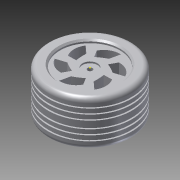
# Autodesk Inventor part: Wheels1
Saved by Autodesk Inventor 2015 (Build 190159000, 159)
## iProperties
Created: 2014-11-04
Part Number: Wheels1
Material: ABS Plastic
Document SubType Name: Modeling
Designer: ah14592
Density: 1.06 g/cm^3
Appearance: Smooth - White
Author: ah14592
Autodesk Inventor part; units mm, degrees
ref_plane "YZ Plane" through (0, 0, 0) normal (1, 0, 0) x (0, 1, 0)
ref_plane "XZ Plane" through (0, 0, 0) normal (0, 1, 0) x (-1, 0, 0)
sketch "Sketch1" plane through (0, 0, 0) normal (0, 1, 0) x (-1, 0, 0)
  line L0 (0, 0) -> (0, 48.3347) construction
  line L1 (-23, 44.2835) -> (-28, 44.2835)
  line L2 (-28, 44.2835) -> (-28, 14.2835)
  line L3 (-28, 14.2835) -> (-23, 14.2835)
  line L4 (-23, 14.2835) -> (-23, 44.2835)
  point P0 (0, 23.2008)
  dimension "d2" = 5
  dimension "d3" = 30
  dimension "d4" = 23
  constraints: 10 end point, 2 parallel, 2 vertical, 1 horizontal, 1 perpendicular, 1 point on line
  measures "d2" distance of L3.end L2.end
  measures "d3" distance of L2.end L1.end
  measures "d4" distance between parallel lines of L4 L0
revolve "Revolution1" add sketch "Sketch1" angle 360 about axis through (0, 0, 0) along (0, 0, 1)
sketch "Sketch7" plane through (0, 0, 44.2835) normal (0, 0, 1) x (1, 0, 0)
  circle A0 centre (0, 0) radius 24
  dimension "d33" = 48
  constraints: 1 centre point, 1 coincident
  measures "d33" diameter of A0
extrude "Extrusion4" add sketch "Sketch7" against normal blind 13
fillet "Fillet4" radius 3 2 edges at (-28, 0, 44.2835) (-28, 0, 14.2835)
sketch "Sketch8" plane through (0, 0, 44.2835) normal (0, 0, 1) x (1, 0, 0)
  circle A0 centre (0, 0) radius 23 projected
  circle A1 centre (0, 0) radius 25 projected
  circle A2 centre (0, 0) radius 28 projected
  circle A3 centre (0, 0) radius 25 projected
  circle A4 centre (0, 0) radius 23
  constraints: 1 centre point, 1 coincident, 1 concentric
fillet "Fillet5" radius 3 1 edges at (-23, 0, 31.2835)
sketch "Sketch9" plane through (0, 0, 44.2835) normal (0, 0, 1) x (1, 0, 0)
  circle A0 centre (0, 0) radius 23 projected
  circle A1 centre (0, 0) radius 20 projected
  circle A2 centre (0, 0) radius 20
  constraints: 1 centre point, 1 coincident, 1 concentric
extrude "Extrusion5" cut sketch "Sketch9" against normal blind 2 contours A1
chamfer "Chamfer1" distance 1 angle 45 1 edges at (-20, 0, 44.2835)
sketch "Sketch10" plane through (0, 0, 42.2835) normal (0, 0, 1) x (1, 0, 0)
  line L0 (-16.9268, -6.6619) -> (-10.5367, -4.6226)
  line L1 (-6.7299, -12.6441) -> (-4.1467, -7.8856)
  arc A0 (-16.9268, -6.6619) -> (-6.7299, -12.6441) centre (-7.1975, -1.7595) ccw
  arc A1 (-10.5367, -4.6226) -> (-4.1467, -7.8856) centre (7.1055, 22.0383) ccw
  point P0 (0, 0)
  constraints: 4 end point, 4 point on circle, 2 centre point
extrude "Extrusion6" cut sketch "Sketch10" against normal through all
pattern_circular "Circular Pattern2" count 6 over 360 about axis through (0, 0, -10) along (0, 0, 1) of "Extrusion6"
sketch "Sketch11" plane through (0, 0, 42.2835) normal (0, 0, 1) x (1, 0, 0)
  point P0 (0, 0)
hole "Hole3" at (0, 0, 44.2835) direction (0, 0, -1) diameter 3.2 end through all counterbore diameter 10 counterbore depth 3
sketch "Sketch12" plane through (0, 0, 31.2835) normal (0, 0, -1) x (-1, 0, 0)
  point P0 (0, 0)
hole "Hole4" at (0, 0, 31.2835) direction (0, 0, 1) diameter 3.2 end through all counterbore diameter 10 counterbore depth 2
sketch "Sketch13" plane through (0, 0, 0) normal (1, 0, 0) x (0, 1, 0)
  line L0 (-28, 17.2835) -> (-28, 41.2835) projected
  line L1 (-28, 39.2835) -> (-27, 39.2835)
  line L2 (-27, 39.2835) -> (-27, 38.2835)
  line L3 (-27, 38.2835) -> (-28, 38.2835)
  line L4 (-28, 38.2835) -> (-28, 39.2835)
  line L5 (-28, 35.7835) -> (-27, 35.7835)
  line L6 (-27, 35.7835) -> (-27, 34.7835)
  line L7 (-27, 34.7835) -> (-28, 34.7835)
  line L8 (-28, 34.7835) -> (-28, 35.7835)
  line L9 (-28, 32.2835) -> (-27, 32.2835)
  line L10 (-27, 32.2835) -> (-27, 31.2835)
  line L11 (-27, 31.2835) -> (-28, 31.2835)
  line L12 (-28, 31.2835) -> (-28, 32.2835)
  line L13 (-28, 41.2835) -> (-28, 17.2835) construction
  arc A0 (-28, 17.2835) -> (-25, 14.2835) centre (-25, 17.2835) ccw construction
  line L14 (-28, 17.2835) -> (28, 17.2835) construction
  line L15 (-28, 29.2835) -> (28, 29.2835) construction
  line L16 (0, -8.8567) -> (0, 53.1402) projected
  point P0 (0, 0)
  dimension "d62" = 1
  dimension "d63" = 1
  dimension "d64" = 1
  dimension "d65" = 1
  dimension "d66" = 1
  dimension "d67" = 1
  dimension "d68" = 10
  dimension "d69" = 2.5
  dimension "d70" = 2.5
  constraints: 28 end point, 6 parallel, 4 horizontal, 4 perpendicular, 1 midpoint, 1 point on line, 1 tangent
  measures "d62" distance of L2.end L3.end
  measures "d63" distance of L1.end L2.end
  measures "d64" distance of L6.end L7.end
  measures "d65" distance of L5.end L6.end
  measures "d66" distance of L10.end L11.end
  measures "d67" distance of L9.end L10.end
  measures "d68" distance between parallel lines of L15 L1
  measures "d69" distance between parallel lines of L9 L7
  measures "d70" distance between parallel lines of L5 L3
revolve "Revolution2" cut sketch "Sketch13" angle 360 about axis through (0, 0, -10) along (0, 0, 1)
ref_plane "Work Plane1" through (0, 0, 29.2835) normal (0, 0, -1) x (-1, 0, 0)
mirror "Mirror1" about plane through (0, 0, 29.2835) normal (0, 0, -1) of "Revolution2"
body "Solid1"
